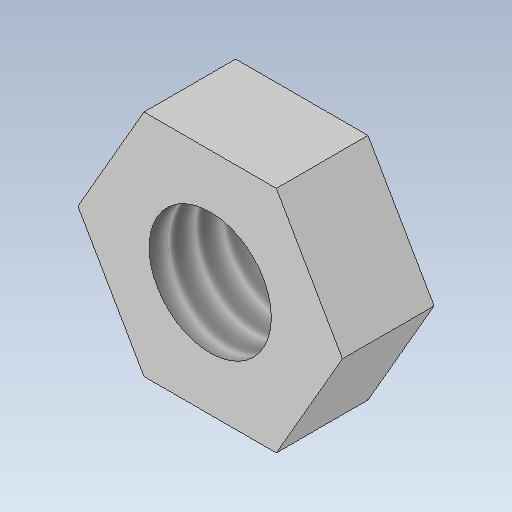
# Autodesk Inventor part: Nut
Saved by Autodesk Inventor 2020 (Build 240168000, 168)
## iProperties
Created: 2018-09-07
Part Number: Nut
Material: 일반
Document SubType Name: Modeling
Designer: Jeong Ji Hoon
Density: 1 g/cm^3
Appearance: 기본값
Author: Jeong Ji Hoon
Autodesk Inventor part; units mm, degrees
ref_plane "YZ Plane" through (0, 0, 0) normal (1, 0, 0) x (0, 1, 0)
ref_plane "XZ Plane" through (0, 0, 0) normal (0, 1, 0) x (-1, 0, 0)
ref_plane "XY Plane" through (0, 0, 0) normal (0, 0, 1) x (1, 0, 0)
sketch "Sketch1" plane through (0, 0, 0) normal (0, 0, 1) x (1, 0, 0)
  line L0 (1.7321, 0) -> (0.866, -1.5)
  line L1 (0.866, -1.5) -> (-0.866, -1.5)
  line L2 (-0.866, -1.5) -> (-1.7321, 0)
  line L3 (-1.7321, 0) -> (-0.866, 1.5)
  line L4 (-0.866, 1.5) -> (0.866, 1.5)
  line L5 (0.866, 1.5) -> (1.7321, 0)
  point P0 (0, 0)
  point P1 (0, 0)
  dimension "d12" = 3
  constraints: 12 end point, 1 coincident, 1 horizontal, 13 other
  measures "d12" distance between parallel lines of L1 L4
extrude "Extrusion1" add sketch "Sketch1" along normal blind 1.2
sketch "Sketch2" plane through (0, 0, 1.2) normal (0, 0, 1) x (1, 0, 0)
  point P0 (0, 0)
  point P1 (0, 0)
  constraints: 1 coincident
hole "Hole1" at (0, 0, 1.2) direction (0, 0, -1) diameter 1.6 end through all
thread "스레드2" size "M1.6x0.35" class "6H" standard "ANSI Metric M Profile" full length
body "Solid1"
